Autodesk Inventor part; units mm, degrees
(part 2 of 2)
sketch "Sketch7" plane through (0, 0, 0) normal (0, 0, -1) x (-1, 0, 0)
  line L0 (-50.8, 47.625) -> (-53.34, 47.625) projected
  line L1 (-53.34, 51.435) -> (-53.34, 47.625) projected
  line L2 (-49.53, 51.435) -> (-53.34, 51.435) projected
  line L3 (-49.53, 51.435) -> (-49.53, 48.895) projected
  line L4 (-50.8, 48.895) -> (-49.53, 48.895) projected
  line L5 (-50.8, 47.625) -> (-50.8, 48.895) projected
  line L6 (-53.34, -10.795) -> (-50.8, -10.795) projected
  line L7 (-50.8, -48.895) -> (-50.8, -10.795) projected
  line L8 (50.8, -48.895) -> (-50.8, -48.895) projected
  line L9 (50.8, 48.895) -> (50.8, -48.895) projected
  line L10 (49.3242, 48.895) -> (50.8, 48.895) projected
  line L11 (49.3242, 48.895) -> (49.3242, 51.435) projected
  line L12 (53.34, 51.435) -> (49.3242, 51.435) projected
  line L13 (53.34, -51.435) -> (53.34, 51.435) projected
  line L14 (-53.34, -51.435) -> (53.34, -51.435) projected
  line L15 (-53.34, -10.795) -> (-53.34, -51.435) projected
  line L16 (53.34, 31.9584) -> (50.8, 31.9584)
  line L17 (50.8, 18.7879) -> (53.34, 18.7879)
  line L18 (53.34, -15.6437) -> (50.8, -15.6437)
  line L19 (50.8, -29.845) -> (53.34, -29.845)
  line L20 (-50.8, -22.6029) -> (-53.34, -22.6029)
  line L21 (-53.34, -38.9912) -> (-50.8, -38.9912)
  point P0 (0, 0)
  constraints: 12 end point, 12 point on line, 6 perpendicular
extrude "Extrusion5" cut sketch "Sketch7" against normal blind 3.81 contours L0 L1 L2 L3 L4 L5 | L20 L7 L21 L15 | L19 L9 L18 L13 | L17 L9 L16 L13
sketch "Sketch8" plane through (0, 0, 19.05) normal (0, 0, -1) x (-1, 0, 0)
  line L0 (11.43, 44.6382) -> (-45.7244, 44.6382) projected
  line L1 (-45.7244, 44.6382) -> (-45.7244, -10.795) projected
  line L2 (-45.7244, -10.795) -> (-49.53, -10.795) projected
  line L3 (-49.53, -10.795) -> (-49.53, -22.225) projected
  line L4 (-49.53, -22.225) -> (-34.29, -22.225) projected
  line L5 (-34.29, -22.225) -> (-34.29, 28.575) projected
  line L6 (-34.29, 28.575) -> (-8.89, 28.575) projected
  line L7 (-8.89, 28.575) -> (-8.89, -22.225) projected
  line L8 (-8.89, -22.225) -> (-1.27, -22.225) projected
  line L9 (-1.27, -22.225) -> (-1.27, 3.937) projected
  line L10 (-1.27, 3.937) -> (49.53, 3.937) projected
  line L11 (49.53, 3.937) -> (49.53, 14.605) projected
  line L12 (49.53, 14.605) -> (11.43, 14.605) projected
  line L13 (11.43, 14.605) -> (11.43, 44.6382) projected
  line L14 (-27.94, -15.875) -> (-27.94, 47.625) projected
  line L15 (49.53, 47.625) -> (-27.94, 47.625) projected
  line L16 (49.53, -22.225) -> (49.53, 47.625) projected
  line L17 (-49.53, -22.225) -> (49.53, -22.225) projected
  line L18 (-49.53, 47.625) -> (-49.53, -22.225) projected
  line L19 (-43.18, 47.625) -> (-49.53, 47.625) projected
  line L20 (-43.18, 47.625) -> (-43.18, -15.875) projected
  line L21 (-43.18, -15.875) -> (-27.94, -15.875) projected
  line L22 (-4.8752, -22.225) -> (10.795, -22.225)
  line L23 (10.795, -22.225) -> (10.795, -12.4001)
  line L24 (10.795, -12.4001) -> (-4.8752, -12.4001)
  line L25 (-4.8752, -12.4001) -> (-4.8752, -22.225)
  point P0 (0, 0)
  constraints: 8 end point, 2 parallel, 1 horizontal, 1 perpendicular, 1 point on line
ref_plane "Work Plane1" through (-49.53, -22.225, 1.778) normal (0, 0, 1) x (1, 0, 0)
extrude "Extrusion6" add sketch "Sketch8" along normal up to surface (17.272 mm away) contours L25 L24 L9 L8 | L24 L23 L17 L9
sketch "Sketch9" plane through (4.8752, -22.225, 1.778) normal (0, 0, -1) x (-1, 0, 0)
  line L0 (0, 9.8249) -> (15.6702, 9.8249) projected
  line L1 (7.8351, 9.8249) -> (10.3751, 9.8249)
  line L2 (10.3751, 9.8249) -> (10.3751, 6.0149)
  line L3 (7.8351, 9.8249) -> (5.2951, 9.8249)
  line L4 (5.2951, 9.8249) -> (5.2951, 6.0149)
  line L5 (5.2951, 6.0149) -> (5.2951, 4.1099)
  line L6 (5.2951, 4.1099) -> (10.3751, 4.1099)
  line L7 (10.3751, 4.1099) -> (10.3751, 6.0149)
  point P0 (4.8752, 22.225)
  dimension "d21" = 2.54
  dimension "d22" = 3.81
  dimension "d23" = 2.54
  dimension "d24" = 1.905
  constraints: 14 end point, 4 perpendicular, 3 point on line, 1 midpoint
  measures "d21" distance of L1.start L1.end
  measures "d22" distance of L1.end L2.end
  measures "d23" distance of L1.start L3.end
  measures "d24" distance of L4.end L5.end
extrude "Extrusion7" cut sketch "Sketch9" against normal blind 2.54
sketch "Sketch10" plane through (0, 0, 19.05) normal (0, 0, -1) x (-1, 0, 0)
  line L0 (50.8, -48.895) -> (50.8, 48.895) projected
  line L1 (50.8, -48.895) -> (44.45, -48.895)
  line L2 (44.45, -48.895) -> (44.45, -42.545)
  line L3 (44.45, -42.545) -> (50.8, -42.545)
  line L4 (50.8, -42.545) -> (50.8, -48.895)
  line L5 (-50.8, -48.895) -> (50.8, -48.895) projected
  line L6 (0, -48.895) -> (0, -34.3816)
  line L7 (-50.8, -48.895) -> (-50.8, 48.895)
  line L8 (-50.8, -48.895) -> (-44.45, -48.895)
  line L9 (-44.45, -48.895) -> (-44.45, -42.545)
  line L10 (-44.45, -42.545) -> (-50.8, -42.545)
  point P0 (0, 0)
  dimension "d27" = 6.35
  dimension "d28" = 6.35
  constraints: 18 end point, 4 symmetric about line, 2 parallel, 1 horizontal, 1 midpoint, 1 perpendicular, 1 vertical
  measures "d27" distance of L2.end L3.end
  measures "d28" distance of L1.end L2.end
extrude "Extrusion8" add sketch "Sketch10" along normal blind 25.4
fillet "Fillet1" radius 3.175 6 edges at (-44.45, -48.895, 9.525) (-50.8, -42.545, 9.525) (44.45, -48.895, 9.525) (50.8, -42.545, 9.525) (44.45, -42.545, 6.35) (-44.45, -42.545, 6.35)
sketch "Sketch11" plane through (0, 0, 19.05) normal (0, 0, -1) x (-1, 0, 0)
  line L0 (-50.8, 47.625) -> (-50.8, -22.6029) projected
  line L1 (50.8, 48.895) -> (-50.8, 48.895)
  line L2 (-50.8, 48.895) -> (-50.8, 44.45)
  line L3 (-50.8, 44.45) -> (50.8, 44.45)
  line L4 (50.8, 44.45) -> (50.8, 48.895)
  point P0 (0, 0)
  dimension "d32" = 4.445
  constraints: 8 end point, 2 parallel, 1 horizontal, 1 perpendicular, 1 point on line
  measures "d32" distance of L2.end L1.end
extrude "Extrusion9" add sketch "Sketch11" along normal blind 15.6972
sketch "Sketch16" plane through (-53.34, -51.435, 22.86) normal (-1, 0, 0) x (0, 0, 1)
  line L0 (-22.86, 83.3934) -> (-19.05, 83.3934) projected
  line L1 (-19.05, 83.3934) -> (-19.05, 70.2229) projected
  line L2 (-19.05, 70.2229) -> (-22.86, 70.2229) projected
  line L3 (-22.86, 70.2229) -> (-22.86, 35.7913) projected
  line L4 (-22.86, 35.7913) -> (-19.05, 35.7913) projected
  line L5 (-19.05, 35.7913) -> (-19.05, 21.59) projected
  line L6 (-19.05, 21.59) -> (-22.86, 21.59) projected
  line L7 (-22.86, 21.59) -> (-22.86, 0) projected
  line L8 (-22.86, 0) -> (0, 0) projected
  line L9 (0, 102.87) -> (0, 0) projected
  line L10 (-22.86, 102.87) -> (0, 102.87) projected
  line L11 (-22.86, 102.87) -> (-22.86, 83.3934) projected
  line L12 (-3.81, 95.885) -> (-19.5072, 95.885) projected
  line L13 (-19.5072, 95.885) -> (-19.5072, 99.06) projected
  line L14 (-19.5072, 99.06) -> (-22.86, 99.06) projected
  line L15 (-22.86, 99.06) -> (-22.86, 28.8321) projected
  line L16 (-22.86, 28.8321) -> (-19.05, 28.8321) projected
  line L17 (-19.05, 28.8321) -> (-19.05, 12.4438) projected
  line L18 (-19.05, 12.4438) -> (-22.86, 12.4438) projected
  line L19 (-22.86, 12.4438) -> (-22.86, 12.065) projected
  line L20 (-3.81, 12.065) -> (-22.86, 12.065) projected
  line L21 (-3.81, 95.885) -> (-3.81, 12.065) projected
  point P0 (-22.86, 51.435)
extrude "Extrusion12" add sketch "Sketch16" against normal up to surface (2.54 mm away) contours L0 L1 L2 L15
sketch "Sketch17" plane through (0, 0, 19.05) normal (0, 0, -1) x (-1, 0, 0)
  arc A0 (-16.256, -45.085) -> (-13.081, -41.91) centre (-16.256, -41.91) ccw projected
  line L0 (-16.256, -45.085) -> (-36.83, -45.085) projected
  arc A1 (-40.005, -41.91) -> (-36.83, -45.085) centre (-36.83, -41.91) ccw projected
  line L1 (-40.005, -41.91) -> (-40.005, -29.083) projected
  arc A2 (-36.83, -25.908) -> (-40.005, -29.083) centre (-36.83, -29.083) ccw projected
  line L2 (-36.83, -25.908) -> (-16.256, -25.908) projected
  arc A3 (-13.081, -29.083) -> (-16.256, -25.908) centre (-16.256, -29.083) ccw projected
  line L3 (-13.081, -29.083) -> (-13.081, -41.91) projected
  line L4 (36.83, -45.085) -> (16.256, -45.085) projected
  arc A4 (13.081, -41.91) -> (16.256, -45.085) centre (16.256, -41.91) ccw projected
  line L5 (13.081, -41.91) -> (13.081, -29.083) projected
  arc A5 (16.256, -25.908) -> (13.081, -29.083) centre (16.256, -29.083) ccw projected
  line L6 (16.256, -25.908) -> (36.83, -25.908) projected
  arc A6 (40.005, -29.083) -> (36.83, -25.908) centre (36.83, -29.083) ccw projected
  line L7 (40.005, -29.083) -> (40.005, -41.91) projected
  arc A7 (36.83, -45.085) -> (40.005, -41.91) centre (36.83, -41.91) ccw projected
  circle A8 centre (-46.863, -35.179) radius 1.27 projected
  circle A9 centre (46.863, -35.179) radius 1.27 projected
  circle A10 centre (-6.223, -35.179) radius 1.27 projected
  circle A11 centre (6.223, -35.179) radius 1.27 projected
  line L8 (10.795, -22.225) -> (-4.8752, -22.225) projected
  line L9 (-4.8752, -22.225) -> (-4.8752, -12.4001) projected
  line L10 (-4.8752, -12.4001) -> (10.795, -12.4001) projected
  line L11 (10.795, -12.4001) -> (10.795, -22.225) projected
  line L12 (50.8, 44.45) -> (-50.8, 44.45) projected
  line L13 (-50.8, 44.45) -> (-50.8, -39.37) projected
  arc A12 (-50.8, -39.37) -> (-47.625, -42.545) centre (-47.625, -39.37) ccw projected
  arc A13 (-44.45, -45.72) -> (-47.625, -42.545) centre (-47.625, -45.72) ccw projected
  arc A14 (-44.45, -45.72) -> (-41.275, -48.895) centre (-41.275, -45.72) ccw projected
  line L14 (-41.275, -48.895) -> (41.275, -48.895) projected
  arc A15 (41.275, -48.895) -> (44.45, -45.72) centre (41.275, -45.72) ccw projected
  arc A16 (47.625, -42.545) -> (44.45, -45.72) centre (47.625, -45.72) ccw projected
  arc A17 (47.625, -42.545) -> (50.8, -39.37) centre (47.625, -39.37) ccw projected
  line L15 (50.8, -39.37) -> (50.8, 44.45) projected
  point P0 (0, 0)
extrude "Extrusion13" add sketch "Sketch17" along normal blind 5.08
sketch "Sketch18" plane through (0, 0, 22.86) normal (0, 0, 1) x (1, 0, 0)
  circle A0 centre (-6.223, -35.179) radius 1.27 projected
  circle A1 centre (6.223, -35.179) radius 1.27 projected
  circle A2 centre (-46.863, -35.179) radius 1.27 projected
  circle A3 centre (46.863, -35.179) radius 1.27 projected
  line L0 (-16.256, -45.085) -> (-36.83, -45.085) projected
  arc A4 (-40.005, -41.91) -> (-36.83, -45.085) centre (-36.83, -41.91) ccw projected
  line L1 (-40.005, -41.91) -> (-40.005, -29.083) projected
  arc A5 (-36.83, -25.908) -> (-40.005, -29.083) centre (-36.83, -29.083) ccw projected
  line L2 (-36.83, -25.908) -> (-16.256, -25.908) projected
  arc A6 (-13.081, -29.083) -> (-16.256, -25.908) centre (-16.256, -29.083) ccw projected
  line L3 (-13.081, -29.083) -> (-13.081, -41.91) projected
  arc A7 (-16.256, -45.085) -> (-13.081, -41.91) centre (-16.256, -41.91) ccw projected
  arc A8 (13.081, -41.91) -> (16.256, -45.085) centre (16.256, -41.91) ccw projected
  line L4 (13.081, -41.91) -> (13.081, -29.083) projected
  arc A9 (16.256, -25.908) -> (13.081, -29.083) centre (16.256, -29.083) ccw projected
  line L5 (16.256, -25.908) -> (36.83, -25.908) projected
  arc A10 (40.005, -29.083) -> (36.83, -25.908) centre (36.83, -29.083) ccw projected
  line L6 (40.005, -29.083) -> (40.005, -41.91) projected
  arc A11 (36.83, -45.085) -> (40.005, -41.91) centre (36.83, -41.91) ccw projected
  line L7 (36.83, -45.085) -> (16.256, -45.085) projected
  line L8 (53.34, 51.435) -> (-53.34, 51.435) projected
  line L9 (-53.34, 51.435) -> (-53.34, -51.435) projected
  line L10 (-53.34, -51.435) -> (53.34, -51.435) projected
  line L11 (53.34, -51.435) -> (53.34, 51.435) projected
  point P0 (0, 0)
extrude "Extrusion14" cut sketch "Sketch18" against normal blind 5.08
sketch "Sketch19" plane through (0, 0, 13.97) normal (0, 0, -1) x (-1, 0, 0)
  line L0 (50.8, 44.45) -> (50.8, -39.37) projected
  line L1 (-50.8, 44.45) -> (50.8, 44.45) projected
  line L2 (-50.8, -39.37) -> (-50.8, 44.45) projected
  arc A0 (-50.8, -39.37) -> (-47.625, -42.545) centre (-47.625, -39.37) ccw projected
  arc A1 (-44.45, -45.72) -> (-47.625, -42.545) centre (-47.625, -45.72) ccw projected
  arc A2 (-44.45, -45.72) -> (-41.275, -48.895) centre (-41.275, -45.72) ccw projected
  line L3 (41.275, -48.895) -> (-41.275, -48.895) projected
  arc A3 (41.275, -48.895) -> (44.45, -45.72) centre (41.275, -45.72) ccw projected
  arc A4 (47.625, -42.545) -> (44.45, -45.72) centre (47.625, -45.72) ccw projected
  arc A5 (47.625, -42.545) -> (50.8, -39.37) centre (47.625, -39.37) ccw projected
  circle A6 centre (-46.863, -35.179) radius 1.27 projected
  circle A7 centre (46.863, -35.179) radius 1.27 projected
  circle A8 centre (-6.223, -35.179) radius 1.27 projected
  circle A9 centre (6.223, -35.179) radius 1.27 projected
  line L4 (-4.8752, -22.225) -> (10.795, -22.225) projected
  line L5 (-4.8752, -12.4001) -> (-4.8752, -22.225) projected
  line L6 (10.795, -12.4001) -> (-4.8752, -12.4001) projected
  line L7 (10.795, -22.225) -> (10.795, -12.4001) projected
  line L8 (40.005, -29.083) -> (40.005, -41.91) projected
  arc A10 (36.83, -45.085) -> (40.005, -41.91) centre (36.83, -41.91) ccw projected
  line L9 (36.83, -45.085) -> (16.256, -45.085) projected
  arc A11 (13.081, -41.91) -> (16.256, -45.085) centre (16.256, -41.91) ccw projected
  line L10 (13.081, -41.91) -> (13.081, -29.083) projected
  arc A12 (16.256, -25.908) -> (13.081, -29.083) centre (16.256, -29.083) ccw projected
  line L11 (16.256, -25.908) -> (36.83, -25.908) projected
  arc A13 (40.005, -29.083) -> (36.83, -25.908) centre (36.83, -29.083) ccw projected
  line L12 (-40.005, -41.91) -> (-40.005, -29.083) projected
  arc A14 (-36.83, -25.908) -> (-40.005, -29.083) centre (-36.83, -29.083) ccw projected
  line L13 (-36.83, -25.908) -> (-16.256, -25.908) projected
  arc A15 (-13.081, -29.083) -> (-16.256, -25.908) centre (-16.256, -29.083) ccw projected
  line L14 (-13.081, -29.083) -> (-13.081, -41.91) projected
  arc A16 (-16.256, -45.085) -> (-13.081, -41.91) centre (-16.256, -41.91) ccw projected
  line L15 (-16.256, -45.085) -> (-36.83, -45.085) projected
  arc A17 (-40.005, -41.91) -> (-36.83, -45.085) centre (-36.83, -41.91) ccw projected
  line L16 (0, -41.275) -> (8.89, -41.275)
  line L17 (8.89, -41.275) -> (8.89, -48.895)
  line L18 (0, -41.275) -> (-8.89, -41.275)
  line L19 (-8.89, -41.275) -> (-8.89, -48.895)
  point P0 (0, 0)
  dimension "d47" = 8.89
  dimension "d48" = 8.89
  constraints: 8 end point, 2 perpendicular, 2 point on line, 1 horizontal
  measures "d47" distance of L16.start L16.end
  measures "d48" distance of L16.start L18.end
extrude "Extrusion15" add sketch "Sketch19" along normal blind 25.4 contours L3 L19 L18 L16 L17
sketch "Sketch20" plane through (-8.89, -48.895, 0) normal (0, -1, 0) x (1, 0, 0)
  line L0 (8.89, 0) -> (8.89, -5.08)
  line L1 (8.89, -5.08) -> (12.7, -5.08)
  line L2 (12.7, -5.08) -> (5.08, -5.08)
  circle A0 centre (12.7, -5.08) radius 1.905
  circle A1 centre (5.08, -5.08) radius 1.905
  dimension "d51" = 5.08
  dimension "d52" = 3.81
  dimension "d53" = 7.62
  dimension "d54" = 3.81
  dimension "d55" = 3.81
  constraints: 6 end point, 2 centre point, 2 coincident, 1 perpendicular, 1 point on line, 1 vertical
  measures "d51" distance of L0.start L0.end
  measures "d52" distance of L0.end L1.end
  measures "d53" distance of L1.end L2.end
  measures "d54" diameter of A0
  measures "d55" diameter of A1
extrude "Extrusion16" cut sketch "Sketch20" against normal blind 25.4
sketch "Sketch21" plane through (-8.89, -48.895, 0) normal (0, -1, 0) x (1, 0, 0)
  line L0 (0, -11.43) -> (17.78, -11.43) projected
  circle A0 centre (5.08, -5.08) radius 1.905 projected
  line L1 (6.985, -5.0834) -> (10.795, -5.0834)
  line L2 (8.89, -5.0834) -> (8.89, 0)
  constraints: 4 end point, 1 horizontal, 1 midpoint, 1 vertical, 2 other
sketch "Sketch22" plane through (0, 0, 17.78) normal (0, 0, 1) x (1, 0, 0)
  line L0 (-53.34, -51.435) -> (-53.34, 51.435) projected
  line L1 (53.34, -51.435) -> (-53.34, -51.435) projected
  line L2 (53.34, 51.435) -> (53.34, -51.435) projected
  line L3 (-53.34, 51.435) -> (53.34, 51.435) projected
  circle A0 centre (-6.223, -35.179) radius 1.27 projected
  circle A1 centre (6.223, -35.179) radius 1.27 projected
  circle A2 centre (-46.863, -35.179) radius 1.27 projected
  circle A3 centre (46.863, -35.179) radius 1.27 projected
  line L4 (36.83, -25.908) -> (16.256, -25.908) projected
  arc A4 (40.005, -29.083) -> (36.83, -25.908) centre (36.83, -29.083) ccw projected
  line L5 (40.005, -41.91) -> (40.005, -29.083) projected
  arc A5 (36.83, -45.085) -> (40.005, -41.91) centre (36.83, -41.91) ccw projected
  line L6 (16.256, -45.085) -> (36.83, -45.085) projected
  arc A6 (13.081, -41.91) -> (16.256, -45.085) centre (16.256, -41.91) ccw projected
  line L7 (13.081, -29.083) -> (13.081, -41.91) projected
  arc A7 (16.256, -25.908) -> (13.081, -29.083) centre (16.256, -29.083) ccw projected
  line L8 (-13.081, -41.91) -> (-13.081, -29.083) projected
  arc A8 (-16.256, -45.085) -> (-13.081, -41.91) centre (-16.256, -41.91) ccw projected
  line L9 (-36.83, -45.085) -> (-16.256, -45.085) projected
  arc A9 (-40.005, -41.91) -> (-36.83, -45.085) centre (-36.83, -41.91) ccw projected
  line L10 (-40.005, -29.083) -> (-40.005, -41.91) projected
  arc A10 (-36.83, -25.908) -> (-40.005, -29.083) centre (-36.83, -29.083) ccw projected
  line L11 (-16.256, -25.908) -> (-36.83, -25.908) projected
  arc A11 (-13.081, -29.083) -> (-16.256, -25.908) centre (-16.256, -29.083) ccw projected
  point P0 (0, 0)
extrude "Extrusion17" add sketch "Sketch22" along normal blind 7.62
sketch "Sketch23" plane through (0, 0, 13.97) normal (0, 0, -1) x (-1, 0, 0)
  line L0 (8.89, -41.275) -> (8.89, -48.895) projected
  line L1 (41.275, -48.895) -> (8.89, -48.895) projected
  arc A0 (41.275, -48.895) -> (44.45, -45.72) centre (41.275, -45.72) ccw projected
  arc A1 (47.625, -42.545) -> (44.45, -45.72) centre (47.625, -45.72) ccw projected
  arc A2 (47.625, -42.545) -> (50.8, -39.37) centre (47.625, -39.37) ccw projected
  line L2 (50.8, 44.45) -> (50.8, -39.37) projected
  line L3 (-50.8, 44.45) -> (50.8, 44.45) projected
  line L4 (-50.8, -39.37) -> (-50.8, 44.45) projected
  arc A3 (-50.8, -39.37) -> (-47.625, -42.545) centre (-47.625, -39.37) ccw projected
  arc A4 (-44.45, -45.72) -> (-47.625, -42.545) centre (-47.625, -45.72) ccw projected
  arc A5 (-44.45, -45.72) -> (-41.275, -48.895) centre (-41.275, -45.72) ccw projected
  line L5 (-8.89, -48.895) -> (-41.275, -48.895) projected
  line L6 (-8.89, -48.895) -> (-8.89, -41.275) projected
  line L7 (-8.89, -41.275) -> (8.89, -41.275) projected
  circle A6 centre (-46.863, -35.179) radius 1.27 projected
  circle A7 centre (46.863, -35.179) radius 1.27 projected
  circle A8 centre (-6.223, -35.179) radius 1.27 projected
  circle A9 centre (6.223, -35.179) radius 1.27 projected
  line L8 (-4.8752, -22.225) -> (10.795, -22.225) projected
  line L9 (-4.8752, -12.4001) -> (-4.8752, -22.225) projected
  line L10 (10.795, -12.4001) -> (-4.8752, -12.4001) projected
  line L11 (10.795, -22.225) -> (10.795, -12.4001) projected
  line L12 (40.005, -29.083) -> (40.005, -41.91) projected
  arc A10 (36.83, -45.085) -> (40.005, -41.91) centre (36.83, -41.91) ccw projected
  line L13 (36.83, -45.085) -> (16.256, -45.085) projected
  arc A11 (13.081, -41.91) -> (16.256, -45.085) centre (16.256, -41.91) ccw projected
  line L14 (13.081, -41.91) -> (13.081, -29.083) projected
  arc A12 (16.256, -25.908) -> (13.081, -29.083) centre (16.256, -29.083) ccw projected
  line L15 (16.256, -25.908) -> (36.83, -25.908) projected
  arc A13 (40.005, -29.083) -> (36.83, -25.908) centre (36.83, -29.083) ccw projected
  line L16 (-40.005, -41.91) -> (-40.005, -29.083) projected
  arc A14 (-36.83, -25.908) -> (-40.005, -29.083) centre (-36.83, -29.083) ccw projected
  line L17 (-36.83, -25.908) -> (-16.256, -25.908) projected
  arc A15 (-13.081, -29.083) -> (-16.256, -25.908) centre (-16.256, -29.083) ccw projected
  line L18 (-13.081, -29.083) -> (-13.081, -41.91) projected
  arc A16 (-16.256, -45.085) -> (-13.081, -41.91) centre (-16.256, -41.91) ccw projected
  line L19 (-16.256, -45.085) -> (-36.83, -45.085) projected
  arc A17 (-40.005, -41.91) -> (-36.83, -45.085) centre (-36.83, -41.91) ccw projected
  point P0 (0, 0)
extrude "Extrusion18" cut sketch "Sketch23" against normal blind 7.62
sketch "Sketch24" plane through (-53.34, 51.435, 0) normal (0, 1, 0) x (1, 0, 0)
  line L0 (104.14, -21.59) -> (2.54, -21.59) projected
  line L1 (102.87, 0) -> (0, 0) projected
  line L2 (53.34, -21.59) -> (53.34, 0)
  line L3 (47.8401, -1.778) -> (52.9201, -1.778) projected
  line L4 (53.34, -10.795) -> (24.0669, -10.795)
  line L5 (24.0669, -10.795) -> (24.0669, -13.335)
  circle A0 centre (24.0669, -13.335) radius 6.985
  line L6 (52.9201, -4.318) -> (47.8401, -4.318) projected
  line L7 (47.8401, -1.778) -> (52.9201, -1.778) projected
  line L8 (47.8401, -1.778) -> (47.8401, -4.318) projected
  line L9 (47.8401, -4.318) -> (52.9201, -4.318) projected
  line L10 (52.9201, -1.778) -> (52.9201, -4.318) projected
  line L11 (47.8401, -1.778) -> (10.2142, -1.778)
  line L12 (47.8401, -4.318) -> (10.4733, -4.318)
  dimension "d63" = 2.54
  dimension "d64" = 13.97
  constraints: 10 end point, 3 horizontal, 2 midpoint, 1 centre point, 1 coincident, 1 perpendicular, 1 vertical
  measures "d63" distance of L4.end L5.end
  measures "d64" diameter of A0
extrude "Extrusion19" cut sketch "Sketch24" against normal blind 7.62 contours A0
sketch "Sketch26" plane through (0, 0, 25.4) normal (0, 0, 1) x (1, 0, 0)
  line L0 (53.34, -51.435) -> (53.34, 51.435) projected
  line L1 (53.34, 51.435) -> (-53.34, 51.435) projected
  line L2 (-53.34, 51.435) -> (-53.34, -51.435) projected
  line L3 (-53.34, -51.435) -> (53.34, -51.435) projected
  circle A0 centre (-6.223, -35.179) radius 1.27 projected
  circle A1 centre (6.223, -35.179) radius 1.27 projected
  circle A2 centre (-46.863, -35.179) radius 1.27 projected
  circle A3 centre (46.863, -35.179) radius 1.27 projected
  arc A4 (-16.256, -45.085) -> (-13.081, -41.91) centre (-16.256, -41.91) ccw projected
  line L4 (-16.256, -45.085) -> (-36.83, -45.085) projected
  arc A5 (-40.005, -41.91) -> (-36.83, -45.085) centre (-36.83, -41.91) ccw projected
  line L5 (-40.005, -41.91) -> (-40.005, -29.083) projected
  arc A6 (-36.83, -25.908) -> (-40.005, -29.083) centre (-36.83, -29.083) ccw projected
  line L6 (-36.83, -25.908) -> (-16.256, -25.908) projected
  arc A7 (-13.081, -29.083) -> (-16.256, -25.908) centre (-16.256, -29.083) ccw projected
  line L7 (-13.081, -29.083) -> (-13.081, -41.91) projected
  arc A8 (40.005, -29.083) -> (36.83, -25.908) centre (36.83, -29.083) ccw projected
  line L8 (40.005, -29.083) -> (40.005, -41.91) projected
  arc A9 (36.83, -45.085) -> (40.005, -41.91) centre (36.83, -41.91) ccw projected
  line L9 (36.83, -45.085) -> (16.256, -45.085) projected
  arc A10 (13.081, -41.91) -> (16.256, -45.085) centre (16.256, -41.91) ccw projected
  line L10 (13.081, -41.91) -> (13.081, -29.083) projected
  arc A11 (16.256, -25.908) -> (13.081, -29.083) centre (16.256, -29.083) ccw projected
  line L11 (16.256, -25.908) -> (36.83, -25.908) projected
  line L12 (55.88, 51.435) -> (55.88, 48.895)
  line L13 (55.88, 48.895) -> (53.34, 48.895)
  line L14 (53.34, 53.975) -> (50.8, 53.975)
  line L15 (50.8, 53.975) -> (50.8, 51.435)
  line L16 (53.34, 53.975) -> (55.88, 53.975)
  line L17 (55.88, 53.975) -> (55.88, 51.2288)
  point P0 (0, 0)
  dimension "d68" = 2.54
  dimension "d69" = 2.54
  dimension "d70" = 2.54
  constraints: 12 end point, 3 point on line, 2 perpendicular, 1 horizontal
  measures "d68" distance of L12.start L12.end
  measures "d69" distance of L0.end L14.start
  measures "d70" distance of L14.start L14.end
extrude "Extrusion20" add sketch "Sketch26" against normal up to surface (21.59 mm away) contours L0 L1 L15 L14 L16 L17 L12 L13
sketch "Sketch27" plane through (0, 0, 25.4) normal (0, 0, 1) x (1, 0, 0)
  line L0 (49.53, 51.435) -> (49.53, 48.895) projected
  line L1 (50.8, 51.435) -> (49.53, 51.435) projected
  line L2 (50.8, 51.435) -> (50.8, 53.975) projected
  line L3 (50.8, 53.975) -> (55.88, 53.975) projected
  line L4 (55.88, 53.975) -> (55.88, 48.895) projected
  line L5 (55.88, 48.895) -> (53.34, 48.895) projected
  line L6 (53.34, 47.625) -> (53.34, 48.895) projected
  line L7 (50.8, 47.625) -> (53.34, 47.625) projected
  line L8 (50.8, 48.895) -> (50.8, 47.625) projected
  line L9 (49.53, 48.895) -> (50.8, 48.895) projected
  line L10 (49.53, 51.435) -> (49.53, 53.975)
  line L11 (49.53, 53.975) -> (50.8, 53.975)
  line L12 (53.34, 47.625) -> (55.88, 47.625)
  line L13 (55.88, 47.625) -> (55.88, 48.895)
  point P0 (0, 0)
  constraints: 8 end point, 2 perpendicular, 1 horizontal, 1 vertical
extrude "Extrusion21" add sketch "Sketch27" against normal up to surface (21.59 mm away) contours L10 L11 L2 L1 | L6 L5 L13 L12
fillet "Fillet2" radius 3.175 2 edges at (53.34, 47.625, 14.605) (49.53, 51.435, 14.605)
sketch "Sketch28" plane through (0, 0, 21.59) normal (0, 0, -1) x (-1, 0, 0)
  line L0 (-36.83, -45.085) -> (-16.256, -45.085) projected
  line L1 (-26.543, -45.085) -> (-12.8905, -45.085)
  line L2 (-12.8905, -45.085) -> (-40.1955, -45.085)
  line L3 (-40.1955, -45.085) -> (-40.1955, -17.78)
  line L4 (-40.1955, -17.78) -> (-12.8905, -17.78)
  line L5 (-12.8905, -17.78) -> (-12.8905, -45.085)
  point P0 (0, 0)
  dimension "d76" = 13.6525
  dimension "d77" = 27.305
  dimension "d78" = 27.305
  dimension "d79" = 27.305
  constraints: 10 end point, 2 perpendicular, 1 collinear, 1 midpoint, 1 point on line
  measures "d76" distance of L1.start L1.end
  measures "d77" distance of L1.end L2.end
  measures "d78" distance of L2.end L3.end
  measures "d79" distance of L3.end L4.end
extrude "Extrusion22" cut sketch "Sketch28" against normal blind 25.4
sketch "Sketch29" plane through (0, 0, 21.59) normal (0, 0, -1) x (-1, 0, 0)
  line L0 (-4.8752, -12.4001) -> (-4.8752, -22.225) projected
  line L1 (10.795, -12.4001) -> (-4.8752, -12.4001) projected
  line L2 (10.795, -22.225) -> (10.795, -12.4001) projected
  line L3 (-4.8752, -22.225) -> (10.795, -22.225) projected
  line L4 (36.83, -25.908) -> (16.256, -25.908) projected
  arc A0 (40.005, -29.083) -> (36.83, -25.908) centre (36.83, -29.083) ccw projected
  line L5 (40.005, -41.91) -> (40.005, -29.083) projected
  arc A1 (36.83, -45.085) -> (40.005, -41.91) centre (36.83, -41.91) ccw projected
  line L6 (16.256, -45.085) -> (36.83, -45.085) projected
  arc A2 (13.081, -41.91) -> (16.256, -45.085) centre (16.256, -41.91) ccw projected
  line L7 (13.081, -29.083) -> (13.081, -41.91) projected
  arc A3 (16.256, -25.908) -> (13.081, -29.083) centre (16.256, -29.083) ccw projected
  line L8 (-12.8905, -45.085) -> (-40.1955, -45.085) projected
  line L9 (-40.1955, -45.085) -> (-40.1955, -17.78) projected
  line L10 (-40.1955, -17.78) -> (-12.8905, -17.78) projected
  line L11 (-12.8905, -17.78) -> (-12.8905, -45.085) projected
  circle A4 centre (6.223, -35.179) radius 1.27 projected
  circle A5 centre (-6.223, -35.179) radius 1.27 projected
  circle A6 centre (46.863, -35.179) radius 1.27 projected
  circle A7 centre (-46.863, -35.179) radius 1.27 projected
  line L12 (8.89, -41.275) -> (-8.89, -41.275) projected
  line L13 (8.89, -48.895) -> (8.89, -41.275) projected
  line L14 (41.275, -48.895) -> (8.89, -48.895) projected
  arc A8 (41.275, -48.895) -> (44.45, -45.72) centre (41.275, -45.72) ccw projected
  arc A9 (47.625, -42.545) -> (44.45, -45.72) centre (47.625, -45.72) ccw projected
  arc A10 (47.625, -42.545) -> (50.8, -39.37) centre (47.625, -39.37) ccw projected
  line L15 (50.8, 44.45) -> (50.8, -39.37) projected
  line L16 (-50.8, 44.45) -> (50.8, 44.45) projected
  line L17 (-50.8, -39.37) -> (-50.8, 44.45) projected
  arc A11 (-50.8, -39.37) -> (-47.625, -42.545) centre (-47.625, -39.37) ccw projected
  arc A12 (-44.45, -45.72) -> (-47.625, -42.545) centre (-47.625, -45.72) ccw projected
  arc A13 (-44.45, -45.72) -> (-41.275, -48.895) centre (-41.275, -45.72) ccw projected
  line L18 (-8.89, -48.895) -> (-41.275, -48.895) projected
  line L19 (-8.89, -41.275) -> (-8.89, -48.895) projected
  point P0 (0, 0)
extrude "Extrusion23" add sketch "Sketch29" against normal up to surface (3.81 mm away) contours A5 | A7
body "Solid1"
